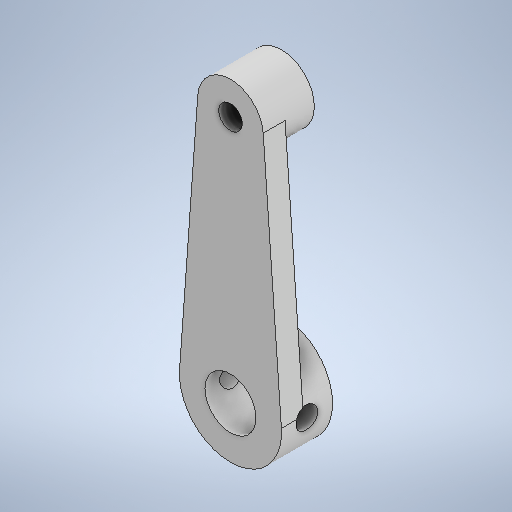
# Autodesk Inventor part: 2072
Saved by Autodesk Inventor 2025.1 (Build 291241000, 241)
## iProperties
Created: 2024-06-10
Part Number: 2072
Material: Generisch
Document SubType Name: Modeling
Designer: ffogue
Density: 1 g/cm^3
Appearance: Vorgabe
Author: ffogue
Autodesk Inventor part; units mm, degrees
note: some values were not read from the file. Chosen so that the rebuilt part matches the saved one: direction of "Bohrung1"; direction of "Bohrung2".
ref_plane "XZ Plane" through (0, 0, 0) normal (0, 1, 0) x (-1, 0, 0)
ref_plane "XY Plane" through (0, 0, 0) normal (0, 0, 1) x (1, 0, 0)
sketch "Skizze1" plane through (0, 0, 0) normal (0, 1, 0) x (-1, 0, 0)
  arc A0 (4.4878, 34.3309) -> (-4.4878, 34.3309) centre (0, 34) ccw
  arc A1 (-6.9811, 0.5147) -> (6.9811, 0.5147) centre (0, 0) ccw
  line L0 (4.4878, 34.3309) -> (6.9811, 0.5147)
  line L1 (-4.4878, 34.3309) -> (-6.9811, 0.5147)
  line L2 (0, 34) -> (0, 0) construction
  dimension "d0" = 34
  dimension "d1" = 14
  dimension "d2" = 9
  constraints: 6 end point, 4 point on circle, 4 tangent, 2 centre point, 1 coincident, 1 vertical, 1 vertical alignment
  measures "d0" distance of L2.end L2.start
  measures "d1" diameter of A1
  measures "d2" diameter of A0
extrude "Extrusion1" add sketch "Skizze1" along normal blind 3
sketch "Skizze2" plane through (0, 3, 0) normal (0, 1, 0) x (1, 0, 0)
  circle A0 centre (0, -34) radius 4.5
  arc A1 (-4.4878, -34.3309) -> (4.4878, -34.3309) centre (0, -34) ccw projected
  circle A2 centre (0, 0) radius 7
  arc A3 (6.9811, -0.5147) -> (-6.9811, -0.5147) centre (0, 0) ccw projected
  dimension "d5" = 9
  dimension "d6" = 14
  constraints: 2 centre point, 2 concentric
  measures "d5" diameter of A0
  measures "d6" diameter of A2
extrude "Extrusion2" add sketch "Skizze2" along normal blind 4
sketch "Skizze3" plane through (0, 7, 34) normal (0, 1, 0) x (1, 0, 0)
  circle A0 centre (0, 0) radius 4.5 projected
  point P0 (0, 34)
  constraints: 1 coincident
hole "Bohrung1" at (0, 7, 34) direction (0, -1, 0) diameter 3.242 depth 7 thread size "M4x0.7" class "6H" standard "ISO Metric profile"
hole "Bohrung2" at (0, 7, 0) direction (0, -1, 0) diameter 7 depth 7
ref_plane "Arbeitsebene1" through (-7, 0, 0) normal (1, 0, 0) x (0, 1, 0)
sketch "Skizze4" plane through (-7, 0, 0) normal (1, 0, 0) x (0, 1, 0)
  line L0 (0, 0.5147) -> (0, 34.3309) projected
  line L1 (0, -7) -> (7, -7) projected
  point P0 (0, 0)
  point P1 (3.5, 0)
  dimension "d24" = 3.5
  constraints: 1 horizontal alignment
  measures "d24" distance from line of L0 point (3.5, 0)
hole "Bohrung3" at (-7, 3.5, 0) direction (1, 0, 0) diameter 3 end through all
